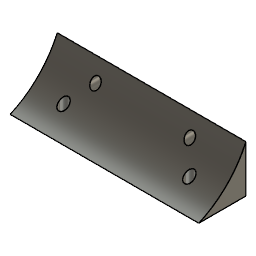
Soporte placa vertical (Autodesk Fusion 360 design; units mm, degrees)
Autodesk Fusion 360 part; units mm, degrees
sketch "Boceto1" plane through (0, 0, 0) normal (1, 0, 0) x (0, 1, 0)
  line L0 (0, 0) -> (-15, 0)
  line L1 (0, 0) -> (0, 15)
  arc A0 (-15, 0) -> (0, 15) centre (-26.7699, 26.7699) ccw
  dimension "d1" = 15
  dimension "d2" = 15
  constraint coincident L0.start L1.start
  constraint horizontal L0
  constraint perpendicular L0 L1
  measures "d1" distance of L0.start L0.end
  measures "d2" distance of L0.start L1.end
extrude "Extruir1" add sketch "Boceto1" along normal blind 60
sketch "Boceto2" plane through (0, 0, 0) normal (0, 1, 0) x (-1, 0, 0)
  line L0 (0, 0) -> (0, 15)
  line L1 (0, 15) -> (-60, 15)
  line L2 (-60, 15) -> (-60, 0)
  line L3 (-60, 0) -> (0, 0)
  circle A0 centre (-45, 10) radius 1.5
  circle A1 centre (-15, 10) radius 1.5
  dimension "d7" = 3
  dimension "d10" = 3
  measures "d7" diameter of A0
  measures "d10" diameter of A1
extrude "Extruir2" cut sketch "Boceto2" against normal blind 4 contours A0 | A1
sketch "Boceto3" plane through (0, 0, 0) normal (0, 0, -1) x (1, 0, 0)
  line L0 (0, 15) -> (0, 0)
  line L1 (0, 0) -> (60, 0)
  line L2 (60, 0) -> (60, 15)
  line L3 (60, 15) -> (0, 15)
  circle A0 centre (10, 8) radius 1.5
  circle A1 centre (50, 8) radius 1.5
  dimension "d17" = 3
  dimension "d18" = 3
  measures "d17" diameter of A0
  measures "d18" diameter of A1
extrude "Extruir3" cut sketch "Boceto3" against normal blind 6 contours A0 | A1
